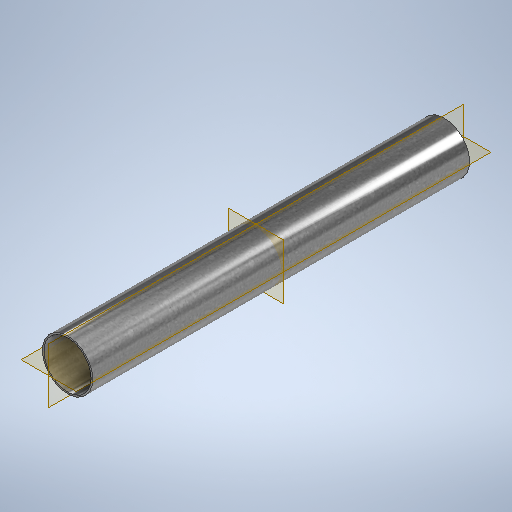
# Autodesk Inventor part: Sessao5_0002_001
Saved by Autodesk Inventor 2025.2 (Build 292293000, 293)
## iProperties
Created: 2025-03-28
Part Number: Sessao5_0002_001
Material: Aço, fundido
Document SubType Name: Modelagem
Designer: lucas
Density: 7.85 g/cm^3
Appearance: Aço galvanizado
Author: lucas
Autodesk Inventor part; units mm, degrees
sketch "Esboço2" plane through (0, 0, 0) normal (0, 0, 1) x (1, 0, 0)
  circle A0 centre (0, 0) radius 50
  circle A1 centre (0, 0) radius 47
  dimension "d6" = 100
  dimension "d7" = 3
  constraints: 2 centre point, 2 coincident
  measures "d6" diameter of A0
  measures "d7" radial gap between concentric circles of A0 A1
extrude "Extrusão1" add sketch "Esboço2" along normal mid plane 750
